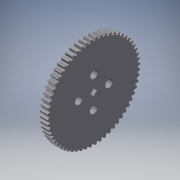
# Autodesk Inventor part: gear60
Saved by Autodesk Inventor 2019 (Build 230136000, 136)
## iProperties
Created: 2019-01-24
Part Number: gear60
Material: Generic
Document SubType Name: Modeling
Designer: Varga Daniel
Density: 1 g/cm^3
Appearance: Default
Author: Varga Daniel
Autodesk Inventor part; units mm, degrees
ref_plane "YZ Plane" through (0, 0, 0) normal (1, 0, 0) x (0, 1, 0)
ref_plane "XZ Plane" through (0, 0, 0) normal (0, 1, 0) x (-1, 0, 0)
ref_plane "XY Plane" through (0, 0, 0) normal (0, 0, 1) x (1, 0, 0)
sketch "Sketch1" plane through (0, 0, 0) normal (1, 0, 0) x (0, 1, 0)
  line L0 (1.5877, 28.5868) -> (1.4918, 28.6064)
  line L1 (1.4918, 28.6064) -> (1.2998, 28.6492)
  line L2 (1.2998, 28.6492) -> (0.9152, 28.7484)
  line L3 (0.9152, 28.7484) -> (0.53, 28.8645)
  line L4 (0.53, 28.8645) -> (0.1446, 28.9962)
  line L5 (0.1446, 28.9962) -> (0.0483, 29.0315)
  line L6 (0.0483, 29.0315) -> (0.0085, 30.0293)
  line L7 (0.0085, 30.0293) -> (0.1018, 30.0721)
  line L8 (0.1018, 30.0721) -> (0.4755, 30.234)
  line L9 (0.4755, 30.234) -> (0.8502, 30.3803)
  line L10 (0.8502, 30.3803) -> (1.2257, 30.5098)
  line L11 (1.2257, 30.5098) -> (1.4137, 30.5678)
  line L12 (1.4137, 30.5678) -> (1.5078, 30.5949)
  line L13 (1.5078, 30.5949) -> (1.521, 31.6473)
  line L14 (1.521, 31.6473) -> (1.4277, 31.6768)
  line L15 (1.4277, 31.6768) -> (1.2412, 31.7395)
  line L16 (1.2412, 31.7395) -> (0.869, 31.8784)
  line L17 (0.869, 31.8784) -> (0.4981, 32.034)
  line L18 (0.4981, 32.034) -> (0.1286, 32.2053)
  line L19 (0.1286, 32.2053) -> (0.0365, 32.2505)
  line L20 (0.0365, 32.2505) -> (0.1012, 33.247)
  line L21 (0.1012, 33.247) -> (0.1985, 33.2798)
  line L22 (0.1985, 33.2798) -> (0.587, 33.4018)
  line L23 (0.587, 33.4018) -> (0.975, 33.5081)
  line L24 (0.975, 33.5081) -> (1.362, 33.5977)
  line L25 (1.362, 33.5977) -> (1.555, 33.6356)
  line L26 (1.555, 33.6356) -> (1.6514, 33.6528)
  line L27 (1.6514, 33.6528) -> (1.7745, 34.6981)
  line L28 (1.7745, 34.6981) -> (1.6848, 34.7372)
  line L29 (1.6848, 34.7372) -> (1.5059, 34.819)
  line L30 (1.5059, 34.819) -> (1.1503, 34.996)
  line L31 (1.1503, 34.996) -> (0.7977, 35.1896)
  line L32 (0.7977, 35.1896) -> (0.4481, 35.3986)
  line L33 (0.4481, 35.3986) -> (0.3612, 35.4531)
  line L34 (0.3612, 35.4531) -> (0.5298, 36.4374)
  line L35 (0.5298, 36.4374) -> (0.6299, 36.4599)
  line L36 (0.6299, 36.4599) -> (1.0291, 36.5406)
  line L37 (1.0291, 36.5406) -> (1.4261, 36.6058)
  line L38 (1.4261, 36.6058) -> (1.8203, 36.6544)
  line L39 (1.8203, 36.6544) -> (2.0162, 36.672)
  line L40 (2.0162, 36.672) -> (2.1138, 36.679)
  line L41 (2.1138, 36.679) -> (2.3456, 37.7056)
  line L42 (2.3456, 37.7056) -> (2.2604, 37.7539)
  line L43 (2.2604, 37.7539) -> (2.0911, 37.8539)
  line L44 (2.0911, 37.8539) -> (1.7559, 38.0672)
  line L45 (1.7559, 38.0672) -> (1.4255, 38.2965)
  line L46 (1.4255, 38.2965) -> (1.0996, 38.5409)
  line L47 (1.0996, 38.5409) -> (1.0189, 38.6042)
  line L48 (1.0189, 38.6042) -> (1.2894, 39.5655)
  line L49 (1.2894, 39.5655) -> (1.3914, 39.5774)
  line L50 (1.3914, 39.5774) -> (1.7968, 39.6159)
  line L51 (1.7968, 39.6159) -> (2.1984, 39.6393)
  line L52 (2.1984, 39.6393) -> (2.5956, 39.6464)
  line L53 (2.5956, 39.6464) -> (2.7923, 39.6434)
  line L54 (2.7923, 39.6434) -> (2.8901, 39.6402)
  line L55 (2.8901, 39.6402) -> (3.2279, 40.637)
  line L56 (3.2279, 40.637) -> (3.1482, 40.6939)
  line L57 (3.1482, 40.6939) -> (2.9903, 40.8111)
  line L58 (2.9903, 40.8111) -> (2.6792, 41.0582)
  line L59 (2.6792, 41.0582) -> (2.3746, 41.3209)
  line L60 (2.3746, 41.3209) -> (2.0761, 41.5979)
  line L61 (2.0761, 41.5979) -> (2.0024, 41.6694)
  line L62 (2.0024, 41.6694) -> (2.372, 42.5971)
  line L63 (2.372, 42.5971) -> (2.4746, 42.5983)
  line L64 (2.4746, 42.5983) -> (2.8818, 42.5942)
  line L65 (2.8818, 42.5942) -> (3.2836, 42.5755)
  line L66 (3.2836, 42.5755) -> (3.6794, 42.541)
  line L67 (3.6794, 42.541) -> (3.8747, 42.5175)
  line L68 (3.8747, 42.5175) -> (3.9716, 42.5041)
  line L69 (3.9716, 42.5041) -> (4.4117, 43.4601)
  line L70 (4.4117, 43.4601) -> (4.3385, 43.525)
  line L71 (4.3385, 43.525) -> (4.1936, 43.6581)
  line L72 (4.1936, 43.6581) -> (3.9101, 43.9364)
  line L73 (3.9101, 43.9364) -> (3.6346, 44.2294)
  line L74 (3.6346, 44.2294) -> (3.3667, 44.5362)
  line L75 (3.3667, 44.5362) -> (3.3008, 44.6149)
  line L76 (3.3008, 44.6149) -> (3.7653, 45.4989)
  line L77 (3.7653, 45.4989) -> (3.8675, 45.4894)
  line L78 (3.8675, 45.4894) -> (4.2721, 45.4428)
  line L79 (4.2721, 45.4428) -> (4.6698, 45.3821)
  line L80 (4.6698, 45.3821) -> (5.0597, 45.3065)
  line L81 (5.0597, 45.3065) -> (5.2515, 45.2626)
  line L82 (5.2515, 45.2626) -> (5.3465, 45.2391)
  line L83 (5.3465, 45.2391) -> (5.8842, 46.1439)
  line L84 (5.8842, 46.1439) -> (5.8181, 46.2161)
  line L85 (5.8181, 46.2161) -> (5.688, 46.3637)
  line L86 (5.688, 46.3637) -> (5.4351, 46.67)
  line L87 (5.4351, 46.67) -> (5.1918, 46.9903)
  line L88 (5.1918, 46.9903) -> (4.9574, 47.3234)
  line L89 (4.9574, 47.3234) -> (4.9002, 47.4086)
  line L90 (4.9002, 47.4086) -> (5.4545, 48.2392)
  line L91 (5.4545, 48.2392) -> (5.5551, 48.219)
  line L92 (5.5551, 48.219) -> (5.9526, 48.1303)
  line L93 (5.9526, 48.1303) -> (6.3418, 48.0285)
  line L94 (6.3418, 48.0285) -> (6.7217, 47.9125)
  line L95 (6.7217, 47.9125) -> (6.9078, 47.8489)
  line L96 (6.9078, 47.8489) -> (6.9999, 47.8156)
  line L97 (6.9999, 47.8156) -> (7.6292, 48.6592)
  line L98 (7.6292, 48.6592) -> (7.571, 48.7379)
  line L99 (7.571, 48.7379) -> (7.457, 48.8982)
  line L100 (7.457, 48.8982) -> (7.2376, 49.2293)
  line L101 (7.2376, 49.2293) -> (7.029, 49.5733)
  line L102 (7.029, 49.5733) -> (6.8307, 49.9291)
  line L103 (6.8307, 49.9291) -> (6.7827, 50.0197)
  line L104 (6.7827, 50.0197) -> (7.4209, 50.7878)
  line L105 (7.4209, 50.7878) -> (7.5188, 50.7573)
  line L106 (7.5188, 50.7573) -> (7.9049, 50.6276)
  line L107 (7.9049, 50.6276) -> (8.2813, 50.4855)
  line L108 (8.2813, 50.4855) -> (8.647, 50.3305)
  line L109 (8.647, 50.3305) -> (8.8255, 50.2478)
  line L110 (8.8255, 50.2478) -> (8.9135, 50.2051)
  line L111 (8.9135, 50.2051) -> (9.6275, 50.9783)
  line L112 (9.6275, 50.9783) -> (9.5779, 51.0627)
  line L113 (9.5779, 51.0627) -> (9.4812, 51.2341)
  line L114 (9.4812, 51.2341) -> (9.2976, 51.5863)
  line L115 (9.2976, 51.5863) -> (9.1261, 51.9502)
  line L116 (9.1261, 51.9502) -> (8.9661, 52.3247)
  line L117 (8.9661, 52.3247) -> (8.9279, 52.4199)
  line L118 (8.9279, 52.4199) -> (9.6428, 53.1171)
  line L119 (9.6428, 53.1171) -> (9.7371, 53.0764)
  line L120 (9.7371, 53.0764) -> (10.1075, 52.9071)
  line L121 (10.1075, 52.9071) -> (10.4669, 52.7265)
  line L122 (10.4669, 52.7265) -> (10.8144, 52.5341)
  line L123 (10.8144, 52.5341) -> (10.9833, 52.4332)
  line L124 (10.9833, 52.4332) -> (11.0664, 52.3814)
  line L125 (11.0664, 52.3814) -> (11.8573, 53.0758)
  line L126 (11.8573, 53.0758) -> (11.8168, 53.1649)
  line L127 (11.8168, 53.1649) -> (11.7386, 53.3454)
  line L128 (11.7386, 53.3454) -> (11.5928, 53.7149)
  line L129 (11.5928, 53.7149) -> (11.4603, 54.0947)
  line L130 (11.4603, 54.0947) -> (11.3404, 54.484)
  line L131 (11.3404, 54.484) -> (11.3123, 54.5827)
  line L132 (11.3123, 54.5827) -> (12.0961, 55.2013)
  line L133 (12.0961, 55.2013) -> (12.1856, 55.151)
  line L134 (12.1856, 55.151) -> (12.5363, 54.9439)
  line L135 (12.5363, 54.9439) -> (12.8749, 54.7267)
  line L136 (12.8749, 54.7267) -> (13.2004, 54.4991)
  line L137 (13.2004, 54.4991) -> (13.3578, 54.381)
  line L138 (13.3578, 54.381) -> (13.435, 54.3209)
  line L139 (13.435, 54.3209) -> (14.2942, 54.9288)
  line L140 (14.2942, 54.9288) -> (14.2632, 55.0216)
  line L141 (14.2632, 55.0216) -> (14.2043, 55.2093)
  line L142 (14.2043, 55.2093) -> (14.0979, 55.592)
  line L143 (14.0979, 55.592) -> (14.0058, 55.9836)
  line L144 (14.0058, 55.9836) -> (13.9272, 56.3832)
  line L145 (13.9272, 56.3832) -> (13.9096, 56.4843)
  line L146 (13.9096, 56.4843) -> (14.7539, 57.0176)
  line L147 (14.7539, 57.0176) -> (14.8376, 56.9583)
  line L148 (14.8376, 56.9583) -> (15.1647, 56.7156)
  line L149 (15.1647, 56.7156) -> (15.4787, 56.4642)
  line L150 (15.4787, 56.4642) -> (15.7786, 56.2038)
  line L151 (15.7786, 56.2038) -> (15.9228, 56.07)
  line L152 (15.9228, 56.07) -> (15.9934, 56.0021)
  line L153 (15.9934, 56.0021) -> (16.9114, 56.5168)
  line L154 (16.9114, 56.5168) -> (16.8902, 56.6124)
  line L155 (16.8902, 56.6124) -> (16.8513, 56.8053)
  line L156 (16.8513, 56.8053) -> (16.7855, 57.197)
  line L157 (16.7855, 57.197) -> (16.7348, 57.596)
  line L158 (16.7348, 57.596) -> (16.6984, 58.0017)
  line L159 (16.6984, 58.0017) -> (16.6914, 58.1041)
  line L160 (16.6914, 58.1041) -> (17.5868, 58.5462)
  line L161 (17.5868, 58.5462) -> (17.6638, 58.4784)
  line L162 (17.6638, 58.4784) -> (17.9638, 58.2029)
  line L163 (17.9638, 58.2029) -> (18.2498, 57.9201)
  line L164 (18.2498, 57.9201) -> (18.5209, 57.6297)
  line L165 (18.5209, 57.6297) -> (18.6503, 57.4815)
  line L166 (18.6503, 57.4815) -> (18.7133, 57.4067)
  line L167 (18.7133, 57.4067) -> (19.6801, 57.8226)
  line L168 (19.6801, 57.8226) -> (19.6691, 57.9199)
  line L169 (19.6691, 57.9199) -> (19.6505, 58.1158)
  line L170 (19.6505, 58.1158) -> (19.626, 58.5122)
  line L171 (19.626, 58.5122) -> (19.6174, 58.9144)
  line L172 (19.6174, 58.9144) -> (19.6235, 59.3216)
  line L173 (19.6235, 59.3216) -> (19.6273, 59.4242)
  line L174 (19.6273, 59.4242) -> (20.564, 59.7703)
  line L175 (20.564, 59.7703) -> (20.6336, 59.6948)
  line L176 (20.6336, 59.6948) -> (20.9031, 59.3895)
  line L177 (20.9031, 59.3895) -> (21.158, 59.0783)
  line L178 (21.158, 59.0783) -> (21.3972, 58.7612)
  line L179 (21.3972, 58.7612) -> (21.5104, 58.6003)
  line L180 (21.5104, 58.6003) -> (21.5653, 58.5192)
  line L181 (21.5653, 58.5192) -> (22.5703, 58.8319)
  line L182 (22.5703, 58.8319) -> (22.5695, 58.9298)
  line L183 (22.5695, 58.9298) -> (22.5714, 59.1265)
  line L184 (22.5714, 59.1265) -> (22.5885, 59.5233)
  line L185 (22.5885, 59.5233) -> (22.622, 59.9242)
  line L186 (22.622, 59.9242) -> (22.6707, 60.3285)
  line L187 (22.6707, 60.3285) -> (22.6851, 60.4301)
  line L188 (22.6851, 60.4301) -> (23.6529, 60.6765)
  line L189 (23.6529, 60.6765) -> (23.7142, 60.5941)
  line L190 (23.7142, 60.5941) -> (23.9503, 60.2623)
  line L191 (23.9503, 60.2623) -> (24.1713, 59.9262)
  line L192 (24.1713, 59.9262) -> (24.376, 59.5858)
  line L193 (24.376, 59.5858) -> (24.4718, 59.4139)
  line L194 (24.4718, 59.4139) -> (24.5179, 59.3276)
  line L195 (24.5179, 59.3276) -> (25.55, 59.5335)
  line L196 (25.55, 59.5335) -> (25.5595, 59.6309)
  line L197 (25.5595, 59.6309) -> (25.582, 59.8263)
  line L198 (25.582, 59.8263) -> (25.6405, 60.2192)
  line L199 (25.6405, 60.2192) -> (25.7157, 60.6144)
  line L200 (25.7157, 60.6144) -> (25.8064, 61.0114)
  line L201 (25.8064, 61.0114) -> (25.8314, 61.111)
  line L202 (25.8314, 61.111) -> (26.8196, 61.2548)
  line L203 (26.8196, 61.2548) -> (26.8719, 61.1665)
  line L204 (26.8719, 61.1665) -> (27.072, 60.8118)
  line L205 (27.072, 60.8118) -> (27.2567, 60.4544)
  line L206 (27.2567, 60.4544) -> (27.4247, 60.0945)
  line L207 (27.4247, 60.0945) -> (27.502, 59.9136)
  line L208 (27.502, 59.9136) -> (27.5388, 59.8229)
  line L209 (27.5388, 59.8229) -> (28.5868, 59.9197)
  line L210 (28.5868, 59.9197) -> (28.6064, 60.0156)
  line L211 (28.6064, 60.0156) -> (28.6493, 60.2076)
  line L212 (28.6493, 60.2076) -> (28.7485, 60.5923)
  line L213 (28.7485, 60.5923) -> (28.8645, 60.9774)
  line L214 (28.8645, 60.9774) -> (28.9963, 61.3628)
  line L215 (28.9963, 61.3628) -> (29.0315, 61.4592)
  line L216 (29.0315, 61.4592) -> (30.0293, 61.4989)
  line L217 (30.0293, 61.4989) -> (30.0722, 61.4057)
  line L218 (30.0722, 61.4057) -> (30.2341, 61.0319)
  line L219 (30.2341, 61.0319) -> (30.3804, 60.6572)
  line L220 (30.3804, 60.6572) -> (30.5099, 60.2817)
  line L221 (30.5099, 60.2817) -> (30.5678, 60.0937)
  line L222 (30.5678, 60.0937) -> (30.595, 59.9997)
  line L223 (30.595, 59.9997) -> (31.6474, 59.9865)
  line L224 (31.6474, 59.9865) -> (31.6769, 60.0798)
  line L225 (31.6769, 60.0798) -> (31.7396, 60.2663)
  line L226 (31.7396, 60.2663) -> (31.8784, 60.6384)
  line L227 (31.8784, 60.6384) -> (32.0341, 61.0093)
  line L228 (32.0341, 61.0093) -> (32.2054, 61.3789)
  line L229 (32.2054, 61.3789) -> (32.2505, 61.471)
  line L230 (32.2505, 61.471) -> (33.247, 61.4062)
  line L231 (33.247, 61.4062) -> (33.2799, 61.309)
  line L232 (33.2799, 61.309) -> (33.4019, 60.9204)
  line L233 (33.4019, 60.9204) -> (33.5082, 60.5325)
  line L234 (33.5082, 60.5325) -> (33.5977, 60.1455)
  line L235 (33.5977, 60.1455) -> (33.6357, 59.9524)
  line L236 (33.6357, 59.9524) -> (33.6529, 59.8561)
  line L237 (33.6529, 59.8561) -> (34.6981, 59.7329)
  line L238 (34.6981, 59.7329) -> (34.7372, 59.8227)
  line L239 (34.7372, 59.8227) -> (34.8191, 60.0016)
  line L240 (34.8191, 60.0016) -> (34.9961, 60.3572)
  line L241 (34.9961, 60.3572) -> (35.1897, 60.7098)
  line L242 (35.1897, 60.7098) -> (35.3986, 61.0594)
  line L243 (35.3986, 61.0594) -> (35.4532, 61.1463)
  line L244 (35.4532, 61.1463) -> (36.4374, 60.9777)
  line L245 (36.4374, 60.9777) -> (36.4599, 60.8776)
  line L246 (36.4599, 60.8776) -> (36.5407, 60.4783)
  line L247 (36.5407, 60.4783) -> (36.6058, 60.0814)
  line L248 (36.6058, 60.0814) -> (36.6544, 59.6872)
  line L249 (36.6544, 59.6872) -> (36.672, 59.4912)
  line L250 (36.672, 59.4912) -> (36.679, 59.3936)
  line L251 (36.679, 59.3936) -> (37.7057, 59.1619)
  line L252 (37.7057, 59.1619) -> (37.754, 59.247)
  line L253 (37.754, 59.247) -> (37.854, 59.4164)
  line L254 (37.854, 59.4164) -> (38.0672, 59.7515)
  line L255 (38.0672, 59.7515) -> (38.2966, 60.082)
  line L256 (38.2966, 60.082) -> (38.541, 60.4078)
  line L257 (38.541, 60.4078) -> (38.6043, 60.4886)
  line L258 (38.6043, 60.4886) -> (39.5656, 60.218)
  line L259 (39.5656, 60.218) -> (39.5775, 60.1161)
  line L260 (39.5775, 60.1161) -> (39.616, 59.7106)
  line L261 (39.616, 59.7106) -> (39.6394, 59.309)
  line L262 (39.6394, 59.309) -> (39.6465, 58.9119)
  line L263 (39.6465, 58.9119) -> (39.6435, 58.7152)
  line L264 (39.6435, 58.7152) -> (39.6403, 58.6174)
  line L265 (39.6403, 58.6174) -> (40.6371, 58.2796)
  line L266 (40.6371, 58.2796) -> (40.694, 58.3592)
  line L267 (40.694, 58.3592) -> (40.8112, 58.5172)
  line L268 (40.8112, 58.5172) -> (41.0583, 58.8282)
  line L269 (41.0583, 58.8282) -> (41.3209, 59.1329)
  line L270 (41.3209, 59.1329) -> (41.598, 59.4314)
  line L271 (41.598, 59.4314) -> (41.6694, 59.5051)
  line L272 (41.6694, 59.5051) -> (42.5971, 59.1355)
  line L273 (42.5971, 59.1355) -> (42.5983, 59.0329)
  line L274 (42.5983, 59.0329) -> (42.5943, 58.6256)
  line L275 (42.5943, 58.6256) -> (42.5755, 58.2238)
  line L276 (42.5755, 58.2238) -> (42.5411, 57.8281)
  line L277 (42.5411, 57.8281) -> (42.5176, 57.6328)
  line L278 (42.5176, 57.6328) -> (42.5042, 57.5358)
  line L279 (42.5042, 57.5358) -> (43.4602, 57.0957)
  line L280 (43.4602, 57.0957) -> (43.5251, 57.169)
  line L281 (43.5251, 57.169) -> (43.6582, 57.3139)
  line L282 (43.6582, 57.3139) -> (43.9364, 57.5974)
  line L283 (43.9364, 57.5974) -> (44.2295, 57.8729)
  line L284 (44.2295, 57.8729) -> (44.5363, 58.1408)
  line L285 (44.5363, 58.1408) -> (44.615, 58.2066)
  line L286 (44.615, 58.2066) -> (45.499, 57.7421)
  line L287 (45.499, 57.7421) -> (45.4895, 57.64)
  line L288 (45.4895, 57.64) -> (45.4428, 57.2353)
  line L289 (45.4428, 57.2353) -> (45.3822, 56.8377)
  line L290 (45.3822, 56.8377) -> (45.3065, 56.4477)
  line L291 (45.3065, 56.4477) -> (45.2627, 56.2559)
  line L292 (45.2627, 56.2559) -> (45.2392, 56.1609)
  line L293 (45.2392, 56.1609) -> (46.144, 55.6233)
  line L294 (46.144, 55.6233) -> (46.2162, 55.6893)
  line L295 (46.2162, 55.6893) -> (46.3637, 55.8195)
  line L296 (46.3637, 55.8195) -> (46.6701, 56.0723)
  line L297 (46.6701, 56.0723) -> (46.9904, 56.3157)
  line L298 (46.9904, 56.3157) -> (47.3235, 56.5501)
  line L299 (47.3235, 56.5501) -> (47.4086, 56.6073)
  line L300 (47.4086, 56.6073) -> (48.2393, 56.053)
  line L301 (48.2393, 56.053) -> (48.2191, 55.9523)
  line L302 (48.2191, 55.9523) -> (48.1304, 55.5548)
  line L303 (48.1304, 55.5548) -> (48.0285, 55.1657)
  line L304 (48.0285, 55.1657) -> (47.9126, 54.7858)
  line L305 (47.9126, 54.7858) -> (47.849, 54.5996)
  line L306 (47.849, 54.5996) -> (47.8156, 54.5076)
  line L307 (47.8156, 54.5076) -> (48.6593, 53.8783)
  line L308 (48.6593, 53.8783) -> (48.738, 53.9364)
  line L309 (48.738, 53.9364) -> (48.8983, 54.0505)
  line L310 (48.8983, 54.0505) -> (49.2294, 54.2699)
  line L311 (49.2294, 54.2699) -> (49.5734, 54.4785)
  line L312 (49.5734, 54.4785) -> (49.9291, 54.6767)
  line L313 (49.9291, 54.6767) -> (50.0198, 54.7248)
  line L314 (50.0198, 54.7248) -> (50.7879, 54.0866)
  line L315 (50.7879, 54.0866) -> (50.7573, 53.9886)
  line L316 (50.7573, 53.9886) -> (50.6276, 53.6026)
  line L317 (50.6276, 53.6026) -> (50.4856, 53.2262)
  line L318 (50.4856, 53.2262) -> (50.3306, 52.8605)
  line L319 (50.3306, 52.8605) -> (50.2479, 52.682)
  line L320 (50.2479, 52.682) -> (50.2051, 52.5939)
  line L321 (50.2051, 52.5939) -> (50.9784, 51.88)
  line L322 (50.9784, 51.88) -> (51.0628, 51.9296)
  line L323 (51.0628, 51.9296) -> (51.2342, 52.0262)
  line L324 (51.2342, 52.0262) -> (51.5864, 52.2098)
  line L325 (51.5864, 52.2098) -> (51.9502, 52.3813)
  line L326 (51.9502, 52.3813) -> (52.3248, 52.5413)
  line L327 (52.3248, 52.5413) -> (52.42, 52.5796)
  line L328 (52.42, 52.5796) -> (53.1172, 51.8646)
  line L329 (53.1172, 51.8646) -> (53.0765, 51.7704)
  line L330 (53.0765, 51.7704) -> (52.9071, 51.4)
  line L331 (52.9071, 51.4) -> (52.7266, 51.0405)
  line L332 (52.7266, 51.0405) -> (52.5342, 50.693)
  line L333 (52.5342, 50.693) -> (52.4332, 50.5242)
  line L334 (52.4332, 50.5242) -> (52.3815, 50.4411)
  line L335 (52.3815, 50.4411) -> (53.0759, 49.6501)
  line L336 (53.0759, 49.6501) -> (53.165, 49.6907)
  line L337 (53.165, 49.6907) -> (53.3455, 49.7689)
  line L338 (53.3455, 49.7689) -> (53.715, 49.9147)
  line L339 (53.715, 49.9147) -> (54.0948, 50.0471)
  line L340 (54.0948, 50.0471) -> (54.484, 50.1671)
  line L341 (54.484, 50.1671) -> (54.5827, 50.1952)
  line L342 (54.5827, 50.1952) -> (55.2014, 49.4113)
  line L343 (55.2014, 49.4113) -> (55.1511, 49.3218)
  line L344 (55.1511, 49.3218) -> (54.944, 48.9712)
  line L345 (54.944, 48.9712) -> (54.7268, 48.6326)
  line L346 (54.7268, 48.6326) -> (54.4991, 48.3071)
  line L347 (54.4991, 48.3071) -> (54.3811, 48.1497)
  line L348 (54.3811, 48.1497) -> (54.321, 48.0725)
  line L349 (54.321, 48.0725) -> (54.9289, 47.2133)
  line L350 (54.9289, 47.2133) -> (55.0217, 47.2443)
  line L351 (55.0217, 47.2443) -> (55.2094, 47.3032)
  line L352 (55.2094, 47.3032) -> (55.5921, 47.4096)
  line L353 (55.5921, 47.4096) -> (55.9837, 47.5016)
  line L354 (55.9837, 47.5016) -> (56.3833, 47.5803)
  line L355 (56.3833, 47.5803) -> (56.4844, 47.5979)
  line L356 (56.4844, 47.5979) -> (57.0177, 46.7536)
  line L357 (57.0177, 46.7536) -> (56.9584, 46.6699)
  line L358 (56.9584, 46.6699) -> (56.7157, 46.3428)
  line L359 (56.7157, 46.3428) -> (56.4643, 46.0287)
  line L360 (56.4643, 46.0287) -> (56.2039, 45.7288)
  line L361 (56.2039, 45.7288) -> (56.07, 45.5847)
  line L362 (56.07, 45.5847) -> (56.0022, 45.5141)
  line L363 (56.0022, 45.5141) -> (56.5169, 44.5961)
  line L364 (56.5169, 44.5961) -> (56.6125, 44.6172)
  line L365 (56.6125, 44.6172) -> (56.8054, 44.6562)
  line L366 (56.8054, 44.6562) -> (57.1971, 44.722)
  line L367 (57.1971, 44.722) -> (57.5961, 44.7726)
  line L368 (57.5961, 44.7726) -> (58.0018, 44.8091)
  line L369 (58.0018, 44.8091) -> (58.1042, 44.8161)
  line L370 (58.1042, 44.8161) -> (58.5463, 43.9207)
  line L371 (58.5463, 43.9207) -> (58.4785, 43.8436)
  line L372 (58.4785, 43.8436) -> (58.203, 43.5437)
  line L373 (58.203, 43.5437) -> (57.9202, 43.2576)
  line L374 (57.9202, 43.2576) -> (57.6298, 42.9866)
  line L375 (57.6298, 42.9866) -> (57.4816, 42.8572)
  line L376 (57.4816, 42.8572) -> (57.4068, 42.7941)
  line L377 (57.4068, 42.7941) -> (57.8227, 41.8273)
  line L378 (57.8227, 41.8273) -> (57.92, 41.8383)
  line L379 (57.92, 41.8383) -> (58.1159, 41.8569)
  line L380 (58.1159, 41.8569) -> (58.5123, 41.8814)
  line L381 (58.5123, 41.8814) -> (58.9145, 41.8901)
  line L382 (58.9145, 41.8901) -> (59.3217, 41.8839)
  line L383 (59.3217, 41.8839) -> (59.4243, 41.8801)
  line L384 (59.4243, 41.8801) -> (59.7704, 40.9434)
  line L385 (59.7704, 40.9434) -> (59.6949, 40.8739)
  line L386 (59.6949, 40.8739) -> (59.3895, 40.6044)
  line L387 (59.3895, 40.6044) -> (59.0784, 40.3495)
  line L388 (59.0784, 40.3495) -> (58.7613, 40.1103)
  line L389 (58.7613, 40.1103) -> (58.6004, 39.997)
  line L390 (58.6004, 39.997) -> (58.5193, 39.9422)
  line L391 (58.5193, 39.9422) -> (58.832, 38.9372)
  line L392 (58.832, 38.9372) -> (58.9298, 38.938)
  line L393 (58.9298, 38.938) -> (59.1266, 38.936)
  line L394 (59.1266, 38.936) -> (59.5234, 38.9189)
  line L395 (59.5234, 38.9189) -> (59.9243, 38.8855)
  line L396 (59.9243, 38.8855) -> (60.3286, 38.8368)
  line L397 (60.3286, 38.8368) -> (60.4302, 38.8223)
  line L398 (60.4302, 38.8223) -> (60.6765, 37.8546)
  line L399 (60.6765, 37.8546) -> (60.5942, 37.7933)
  line L400 (60.5942, 37.7933) -> (60.2624, 37.5572)
  line L401 (60.2624, 37.5572) -> (59.9262, 37.3362)
  line L402 (59.9262, 37.3362) -> (59.5859, 37.1314)
  line L403 (59.5859, 37.1314) -> (59.414, 37.0357)
  line L404 (59.414, 37.0357) -> (59.3277, 36.9895)
  line L405 (59.3277, 36.9895) -> (59.5336, 35.9574)
  line L406 (59.5336, 35.9574) -> (59.631, 35.9479)
  line L407 (59.631, 35.9479) -> (59.8264, 35.9254)
  line L408 (59.8264, 35.9254) -> (60.2193, 35.8669)
  line L409 (60.2193, 35.8669) -> (60.6145, 35.7918)
  line L410 (60.6145, 35.7918) -> (61.0115, 35.7011)
  line L411 (61.0115, 35.7011) -> (61.1111, 35.6761)
  line L412 (61.1111, 35.6761) -> (61.2549, 34.6879)
  line L413 (61.2549, 34.6879) -> (61.166, 34.6351)
  line L414 (61.166, 34.6351) -> (60.8112, 34.435)
  line L415 (60.8112, 34.435) -> (60.4539, 34.2504)
  line L416 (60.4539, 34.2504) -> (60.0941, 34.0824)
  line L417 (60.0941, 34.0824) -> (59.9131, 34.0051)
  line L418 (59.9131, 34.0051) -> (59.8224, 33.9683)
  line L419 (59.8224, 33.9683) -> (59.9193, 32.9203)
  line L420 (59.9193, 32.9203) -> (60.016, 32.9005)
  line L421 (60.016, 32.9005) -> (60.208, 32.8577)
  line L422 (60.208, 32.8577) -> (60.5926, 32.7585)
  line L423 (60.5926, 32.7585) -> (60.9778, 32.6424)
  line L424 (60.9778, 32.6424) -> (61.3632, 32.5107)
  line L425 (61.3632, 32.5107) -> (61.4595, 32.4754)
  line L426 (61.4595, 32.4754) -> (61.4992, 31.4784)
  line L427 (61.4992, 31.4784) -> (61.4056, 31.4354)
  line L428 (61.4056, 31.4354) -> (61.0319, 31.2735)
  line L429 (61.0319, 31.2735) -> (60.6572, 31.1272)
  line L430 (60.6572, 31.1272) -> (60.2817, 30.9977)
  line L431 (60.2817, 30.9977) -> (60.0937, 30.9398)
  line L432 (60.0937, 30.9398) -> (59.9996, 30.9126)
  line L433 (59.9996, 30.9126) -> (59.9864, 29.8602)
  line L434 (59.9864, 29.8602) -> (60.0797, 29.8307)
  line L435 (60.0797, 29.8307) -> (60.2662, 29.768)
  line L436 (60.2662, 29.768) -> (60.6384, 29.6292)
  line L437 (60.6384, 29.6292) -> (61.0093, 29.4735)
  line L438 (61.0093, 29.4735) -> (61.3788, 29.3022)
  line L439 (61.3788, 29.3022) -> (61.4709, 29.2571)
  line L440 (61.4709, 29.2571) -> (61.4062, 28.2615)
  line L441 (61.4062, 28.2615) -> (61.3094, 28.2287)
  line L442 (61.3094, 28.2287) -> (60.9208, 28.1068)
  line L443 (60.9208, 28.1068) -> (60.5328, 28.0004)
  line L444 (60.5328, 28.0004) -> (60.1458, 27.9109)
  line L445 (60.1458, 27.9109) -> (59.9528, 27.8729)
  line L446 (59.9528, 27.8729) -> (59.8564, 27.8557)
  line L447 (59.8564, 27.8557) -> (59.7333, 26.8105)
  line L448 (59.7333, 26.8105) -> (59.823, 26.7714)
  line L449 (59.823, 26.7714) -> (60.0019, 26.6896)
  line L450 (60.0019, 26.6896) -> (60.3575, 26.5126)
  line L451 (60.3575, 26.5126) -> (60.7101, 26.319)
  line L452 (60.7101, 26.319) -> (61.0597, 26.11)
  line L453 (61.0597, 26.11) -> (61.1467, 26.0555)
  line L454 (61.1467, 26.0555) -> (60.9781, 25.0712)
  line L455 (60.9781, 25.0712) -> (60.8779, 25.0487)
  line L456 (60.8779, 25.0487) -> (60.4787, 24.968)
  line L457 (60.4787, 24.968) -> (60.0818, 24.9028)
  line L458 (60.0818, 24.9028) -> (59.6876, 24.8542)
  line L459 (59.6876, 24.8542) -> (59.4916, 24.8366)
  line L460 (59.4916, 24.8366) -> (59.394, 24.8296)
  line L461 (59.394, 24.8296) -> (59.1622, 23.8029)
  line L462 (59.1622, 23.8029) -> (59.2474, 23.7547)
  line L463 (59.2474, 23.7547) -> (59.4168, 23.6546)
  line L464 (59.4168, 23.6546) -> (59.7519, 23.4414)
  line L465 (59.7519, 23.4414) -> (60.0823, 23.212)
  line L466 (60.0823, 23.212) -> (60.4082, 22.9676)
  line L467 (60.4082, 22.9676) -> (60.4889, 22.9043)
  line L468 (60.4889, 22.9043) -> (60.2184, 21.9431)
  line L469 (60.2184, 21.9431) -> (60.1165, 21.9311)
  line L470 (60.1165, 21.9311) -> (59.711, 21.8926)
  line L471 (59.711, 21.8926) -> (59.3094, 21.8693)
  line L472 (59.3094, 21.8693) -> (58.9123, 21.8622)
  line L473 (58.9123, 21.8622) -> (58.7156, 21.8651)
  line L474 (58.7156, 21.8651) -> (58.6175, 21.8684)
  line L475 (58.6175, 21.8684) -> (58.2797, 20.8716)
  line L476 (58.2797, 20.8716) -> (58.3594, 20.8147)
  line L477 (58.3594, 20.8147) -> (58.5174, 20.6974)
  line L478 (58.5174, 20.6974) -> (58.8284, 20.4504)
  line L479 (58.8284, 20.4504) -> (59.133, 20.1877)
  line L480 (59.133, 20.1877) -> (59.4316, 19.9106)
  line L481 (59.4316, 19.9106) -> (59.5052, 19.8392)
  line L482 (59.5052, 19.8392) -> (59.1357, 18.9115)
  line L483 (59.1357, 18.9115) -> (59.0331, 18.9103)
  line L484 (59.0331, 18.9103) -> (58.6258, 18.9143)
  line L485 (58.6258, 18.9143) -> (58.224, 18.9331)
  line L486 (58.224, 18.9331) -> (57.8283, 18.9675)
  line L487 (57.8283, 18.9675) -> (57.6329, 18.991)
  line L488 (57.6329, 18.991) -> (57.536, 19.0045)
  line L489 (57.536, 19.0045) -> (57.0955, 18.0476)
  line L490 (57.0955, 18.0476) -> (57.1691, 17.9823)
  line L491 (57.1691, 17.9823) -> (57.314, 17.8493)
  line L492 (57.314, 17.8493) -> (57.5975, 17.571)
  line L493 (57.5975, 17.571) -> (57.873, 17.278)
  line L494 (57.873, 17.278) -> (58.1409, 16.9712)
  line L495 (58.1409, 16.9712) -> (58.2067, 16.8925)
  line L496 (58.2067, 16.8925) -> (57.7422, 16.0085)
  line L497 (57.7422, 16.0085) -> (57.6401, 16.018)
  line L498 (57.6401, 16.018) -> (57.2355, 16.0646)
  line L499 (57.2355, 16.0646) -> (56.8378, 16.1253)
  line L500 (56.8378, 16.1253) -> (56.4479, 16.2009)
  line L501 (56.4479, 16.2009) -> (56.2561, 16.2447)
  line L502 (56.2561, 16.2447) -> (56.161, 16.2682)
  line L503 (56.161, 16.2682) -> (55.6234, 15.3635)
  line L504 (55.6234, 15.3635) -> (55.6895, 15.2912)
  line L505 (55.6895, 15.2912) -> (55.8196, 15.1437)
  line L506 (55.8196, 15.1437) -> (56.0724, 14.8374)
  line L507 (56.0724, 14.8374) -> (56.3158, 14.5171)
  line L508 (56.3158, 14.5171) -> (56.5502, 14.184)
  line L509 (56.5502, 14.184) -> (56.6074, 14.0988)
  line L510 (56.6074, 14.0988) -> (56.0531, 13.2682)
  line L511 (56.0531, 13.2682) -> (55.9525, 13.2884)
  line L512 (55.9525, 13.2884) -> (55.5549, 13.377)
  line L513 (55.5549, 13.377) -> (55.1658, 13.4789)
  line L514 (55.1658, 13.4789) -> (54.7859, 13.5949)
  line L515 (54.7859, 13.5949) -> (54.5997, 13.6585)
  line L516 (54.5997, 13.6585) -> (54.5077, 13.6918)
  line L517 (54.5077, 13.6918) -> (53.8784, 12.8482)
  line L518 (53.8784, 12.8482) -> (53.9366, 12.7695)
  line L519 (53.9366, 12.7695) -> (54.0506, 12.6092)
  line L520 (54.0506, 12.6092) -> (54.27, 12.2781)
  line L521 (54.27, 12.2781) -> (54.4786, 11.9341)
  line L522 (54.4786, 11.9341) -> (54.6769, 11.5783)
  line L523 (54.6769, 11.5783) -> (54.7249, 11.4876)
  line L524 (54.7249, 11.4876) -> (54.0867, 10.7196)
  line L525 (54.0867, 10.7196) -> (53.9888, 10.7501)
  line L526 (53.9888, 10.7501) -> (53.6027, 10.8798)
  line L527 (53.6027, 10.8798) -> (53.2263, 11.0218)
  line L528 (53.2263, 11.0218) -> (52.8606, 11.1769)
  line L529 (52.8606, 11.1769) -> (52.6821, 11.2596)
  line L530 (52.6821, 11.2596) -> (52.5941, 11.3023)
  line L531 (52.5941, 11.3023) -> (51.8801, 10.529)
  line L532 (51.8801, 10.529) -> (51.9297, 10.4447)
  line L533 (51.9297, 10.4447) -> (52.0264, 10.2733)
  line L534 (52.0264, 10.2733) -> (52.21, 9.9211)
  line L535 (52.21, 9.9211) -> (52.3815, 9.5572)
  line L536 (52.3815, 9.5572) -> (52.5414, 9.1827)
  line L537 (52.5414, 9.1827) -> (52.5797, 9.0874)
  line L538 (52.5797, 9.0874) -> (51.8648, 8.3903)
  line L539 (51.8648, 8.3903) -> (51.7705, 8.4309)
  line L540 (51.7705, 8.4309) -> (51.4001, 8.6003)
  line L541 (51.4001, 8.6003) -> (51.0407, 8.7809)
  line L542 (51.0407, 8.7809) -> (50.6932, 8.9733)
  line L543 (50.6932, 8.9733) -> (50.5243, 9.0742)
  line L544 (50.5243, 9.0742) -> (50.4412, 9.1259)
  line L545 (50.4412, 9.1259) -> (49.6503, 8.4316)
  line L546 (49.6503, 8.4316) -> (49.6908, 8.3425)
  line L547 (49.6908, 8.3425) -> (49.769, 8.162)
  line L548 (49.769, 8.162) -> (49.9148, 7.7925)
  line L549 (49.9148, 7.7925) -> (50.0473, 7.4126)
  line L550 (50.0473, 7.4126) -> (50.1672, 7.0234)
  line L551 (50.1672, 7.0234) -> (50.1953, 6.9247)
  line L552 (50.1953, 6.9247) -> (49.4114, 6.3061)
  line L553 (49.4114, 6.3061) -> (49.322, 6.3563)
  line L554 (49.322, 6.3563) -> (48.9713, 6.5635)
  line L555 (48.9713, 6.5635) -> (48.6327, 6.7806)
  line L556 (48.6327, 6.7806) -> (48.3072, 7.0083)
  line L557 (48.3072, 7.0083) -> (48.1498, 7.1264)
  line L558 (48.1498, 7.1264) -> (48.0726, 7.1865)
  line L559 (48.0726, 7.1865) -> (47.2134, 6.5786)
  line L560 (47.2134, 6.5786) -> (47.2444, 6.4857)
  line L561 (47.2444, 6.4857) -> (47.3033, 6.298)
  line L562 (47.3033, 6.298) -> (47.4097, 5.9153)
  line L563 (47.4097, 5.9153) -> (47.5018, 5.5238)
  line L564 (47.5018, 5.5238) -> (47.5804, 5.1241)
  line L565 (47.5804, 5.1241) -> (47.598, 5.023)
  line L566 (47.598, 5.023) -> (46.7537, 4.4897)
  line L567 (46.7537, 4.4897) -> (46.67, 4.5491)
  line L568 (46.67, 4.5491) -> (46.3429, 4.7918)
  line L569 (46.3429, 4.7918) -> (46.0289, 5.0431)
  line L570 (46.0289, 5.0431) -> (45.729, 5.3036)
  line L571 (45.729, 5.3036) -> (45.5848, 5.4374)
  line L572 (45.5848, 5.4374) -> (45.5142, 5.5053)
  line L573 (45.5142, 5.5053) -> (44.5962, 4.9905)
  line L574 (44.5962, 4.9905) -> (44.6173, 4.8949)
  line L575 (44.6173, 4.8949) -> (44.6563, 4.7021)
  line L576 (44.6563, 4.7021) -> (44.7221, 4.3104)
  line L577 (44.7221, 4.3104) -> (44.7728, 3.9113)
  line L578 (44.7728, 3.9113) -> (44.8092, 3.5057)
  line L579 (44.8092, 3.5057) -> (44.8162, 3.4033)
  line L580 (44.8162, 3.4033) -> (43.9208, 2.9611)
  line L581 (43.9208, 2.9611) -> (43.8437, 3.0289)
  line L582 (43.8437, 3.0289) -> (43.5438, 3.3045)
  line L583 (43.5438, 3.3045) -> (43.2577, 3.5873)
  line L584 (43.2577, 3.5873) -> (42.9867, 3.8776)
  line L585 (42.9867, 3.8776) -> (42.8573, 4.0258)
  line L586 (42.8573, 4.0258) -> (42.7942, 4.1007)
  line L587 (42.7942, 4.1007) -> (41.8274, 3.6847)
  line L588 (41.8274, 3.6847) -> (41.8384, 3.5875)
  line L589 (41.8384, 3.5875) -> (41.857, 3.3916)
  line L590 (41.857, 3.3916) -> (41.8815, 2.9952)
  line L591 (41.8815, 2.9952) -> (41.8902, 2.593)
  line L592 (41.8902, 2.593) -> (41.884, 2.1857)
  line L593 (41.884, 2.1857) -> (41.8802, 2.0832)
  line L594 (41.8802, 2.0832) -> (40.9435, 1.7371)
  line L595 (40.9435, 1.7371) -> (40.874, 1.8125)
  line L596 (40.874, 1.8125) -> (40.6045, 2.1179)
  line L597 (40.6045, 2.1179) -> (40.3496, 2.4291)
  line L598 (40.3496, 2.4291) -> (40.1104, 2.7462)
  line L599 (40.1104, 2.7462) -> (39.9972, 2.9071)
  line L600 (39.9972, 2.9071) -> (39.9423, 2.9881)
  line L601 (39.9423, 2.9881) -> (38.9373, 2.6755)
  line L602 (38.9373, 2.6755) -> (38.9381, 2.5776)
  line L603 (38.9381, 2.5776) -> (38.9361, 2.3809)
  line L604 (38.9361, 2.3809) -> (38.919, 1.984)
  line L605 (38.919, 1.984) -> (38.8856, 1.5832)
  line L606 (38.8856, 1.5832) -> (38.8369, 1.1788)
  line L607 (38.8369, 1.1788) -> (38.8224, 1.0772)
  line L608 (38.8224, 1.0772) -> (37.8547, 0.8309)
  line L609 (37.8547, 0.8309) -> (37.7934, 0.9132)
  line L610 (37.7934, 0.9132) -> (37.5573, 1.2451)
  line L611 (37.5573, 1.2451) -> (37.3363, 1.5812)
  line L612 (37.3363, 1.5812) -> (37.1316, 1.9216)
  line L613 (37.1316, 1.9216) -> (37.0358, 2.0934)
  line L614 (37.0358, 2.0934) -> (36.9897, 2.1798)
  line L615 (36.9897, 2.1798) -> (35.9575, 1.9739)
  line L616 (35.9575, 1.9739) -> (35.9481, 1.8765)
  line L617 (35.9481, 1.8765) -> (35.9255, 1.681)
  line L618 (35.9255, 1.681) -> (35.8671, 1.2882)
  line L619 (35.8671, 1.2882) -> (35.7919, 0.893)
  line L620 (35.7919, 0.893) -> (35.7012, 0.4959)
  line L621 (35.7012, 0.4959) -> (35.6762, 0.3964)
  line L622 (35.6762, 0.3964) -> (34.688, 0.2526)
  line L623 (34.688, 0.2526) -> (34.6357, 0.3408)
  line L624 (34.6357, 0.3408) -> (34.4355, 0.6956)
  line L625 (34.4355, 0.6956) -> (34.2509, 1.053)
  line L626 (34.2509, 1.053) -> (34.0828, 1.4129)
  line L627 (34.0828, 1.4129) -> (34.0056, 1.5938)
  line L628 (34.0056, 1.5938) -> (33.9687, 1.6845)
  line L629 (33.9687, 1.6845) -> (32.9207, 1.5876)
  line L630 (32.9207, 1.5876) -> (32.9011, 1.4917)
  line L631 (32.9011, 1.4917) -> (32.8583, 1.2997)
  line L632 (32.8583, 1.2997) -> (32.7591, 0.9151)
  line L633 (32.7591, 0.9151) -> (32.643, 0.5299)
  line L634 (32.643, 0.5299) -> (32.5113, 0.1445)
  line L635 (32.5113, 0.1445) -> (32.476, 0.0482)
  line L636 (32.476, 0.0482) -> (31.4782, 0.0084)
  line L637 (31.4782, 0.0084) -> (31.4354, 0.1017)
  line L638 (31.4354, 0.1017) -> (31.2735, 0.4754)
  line L639 (31.2735, 0.4754) -> (31.1272, 0.8501)
  line L640 (31.1272, 0.8501) -> (30.9977, 1.2256)
  line L641 (30.9977, 1.2256) -> (30.9397, 1.4136)
  line L642 (30.9397, 1.4136) -> (30.9126, 1.5077)
  line L643 (30.9126, 1.5077) -> (29.8602, 1.5209)
  line L644 (29.8602, 1.5209) -> (29.8307, 1.4276)
  line L645 (29.8307, 1.4276) -> (29.768, 1.2411)
  line L646 (29.768, 1.2411) -> (29.6291, 0.8689)
  line L647 (29.6291, 0.8689) -> (29.4735, 0.498)
  line L648 (29.4735, 0.498) -> (29.3022, 0.1285)
  line L649 (29.3022, 0.1285) -> (29.257, 0.0364)
  line L650 (29.257, 0.0364) -> (28.2605, 0.1011)
  line L651 (28.2605, 0.1011) -> (28.2277, 0.1984)
  line L652 (28.2277, 0.1984) -> (28.1057, 0.587)
  line L653 (28.1057, 0.587) -> (27.9994, 0.9749)
  line L654 (27.9994, 0.9749) -> (27.9098, 1.3619)
  line L655 (27.9098, 1.3619) -> (27.8718, 1.5549)
  line L656 (27.8718, 1.5549) -> (27.8547, 1.6513)
  line L657 (27.8547, 1.6513) -> (26.8094, 1.7744)
  line L658 (26.8094, 1.7744) -> (26.7703, 1.6847)
  line L659 (26.7703, 1.6847) -> (26.6885, 1.5058)
  line L660 (26.6885, 1.5058) -> (26.5115, 1.1502)
  line L661 (26.5115, 1.1502) -> (26.3179, 0.7976)
  line L662 (26.3179, 0.7976) -> (26.1089, 0.448)
  line L663 (26.1089, 0.448) -> (26.0544, 0.3611)
  line L664 (26.0544, 0.3611) -> (25.0701, 0.5297)
  line L665 (25.0701, 0.5297) -> (25.0476, 0.6298)
  line L666 (25.0476, 0.6298) -> (24.9669, 1.029)
  line L667 (24.9669, 1.029) -> (24.9017, 1.426)
  line L668 (24.9017, 1.426) -> (24.8531, 1.8202)
  line L669 (24.8531, 1.8202) -> (24.8355, 2.0161)
  line L670 (24.8355, 2.0161) -> (24.8285, 2.1138)
  line L671 (24.8285, 2.1138) -> (23.8019, 2.3455)
  line L672 (23.8019, 2.3455) -> (23.7536, 2.2603)
  line L673 (23.7536, 2.2603) -> (23.6535, 2.091)
  line L674 (23.6535, 2.091) -> (23.4403, 1.7558)
  line L675 (23.4403, 1.7558) -> (23.2109, 1.4254)
  line L676 (23.2109, 1.4254) -> (22.9666, 1.0996)
  line L677 (22.9666, 1.0996) -> (22.9032, 1.0188)
  line L678 (22.9032, 1.0188) -> (21.942, 1.2894)
  line L679 (21.942, 1.2894) -> (21.9301, 1.3913)
  line L680 (21.9301, 1.3913) -> (21.8915, 1.7967)
  line L681 (21.8915, 1.7967) -> (21.8682, 2.1983)
  line L682 (21.8682, 2.1983) -> (21.8611, 2.5955)
  line L683 (21.8611, 2.5955) -> (21.8641, 2.7922)
  line L684 (21.8641, 2.7922) -> (21.8673, 2.89)
  line L685 (21.8673, 2.89) -> (20.8705, 3.2278)
  line L686 (20.8705, 3.2278) -> (20.8136, 3.1481)
  line L687 (20.8136, 3.1481) -> (20.6964, 2.9902)
  line L688 (20.6964, 2.9902) -> (20.4493, 2.6791)
  line L689 (20.4493, 2.6791) -> (20.1866, 2.3745)
  line L690 (20.1866, 2.3745) -> (19.9095, 2.076)
  line L691 (19.9095, 2.076) -> (19.8381, 2.0023)
  line L692 (19.8381, 2.0023) -> (18.9104, 2.3719)
  line L693 (18.9104, 2.3719) -> (18.9092, 2.4745)
  line L694 (18.9092, 2.4745) -> (18.9133, 2.8817)
  line L695 (18.9133, 2.8817) -> (18.932, 3.2836)
  line L696 (18.932, 3.2836) -> (18.9664, 3.6793)
  line L697 (18.9664, 3.6793) -> (18.99, 3.8746)
  line L698 (18.99, 3.8746) -> (19.0034, 3.9716)
  line L699 (19.0034, 3.9716) -> (18.0473, 4.4116)
  line L700 (18.0473, 4.4116) -> (17.9824, 4.3384)
  line L701 (17.9824, 4.3384) -> (17.8493, 4.1935)
  line L702 (17.8493, 4.1935) -> (17.5711, 3.91)
  line L703 (17.5711, 3.91) -> (17.278, 3.6345)
  line L704 (17.278, 3.6345) -> (16.9713, 3.3666)
  line L705 (16.9713, 3.3666) -> (16.8925, 3.3008)
  line L706 (16.8925, 3.3008) -> (16.0085, 3.7653)
  line L707 (16.0085, 3.7653) -> (16.0181, 3.8674)
  line L708 (16.0181, 3.8674) -> (16.0647, 4.2721)
  line L709 (16.0647, 4.2721) -> (16.1254, 4.6697)
  line L710 (16.1254, 4.6697) -> (16.201, 5.0596)
  line L711 (16.201, 5.0596) -> (16.2448, 5.2514)
  line L712 (16.2448, 5.2514) -> (16.2683, 5.3465)
  line L713 (16.2683, 5.3465) -> (15.3635, 5.8841)
  line L714 (15.3635, 5.8841) -> (15.2913, 5.8181)
  line L715 (15.2913, 5.8181) -> (15.1438, 5.6879)
  line L716 (15.1438, 5.6879) -> (14.8374, 5.4351)
  line L717 (14.8374, 5.4351) -> (14.5172, 5.1917)
  line L718 (14.5172, 5.1917) -> (14.1841, 4.9573)
  line L719 (14.1841, 4.9573) -> (14.0989, 4.9001)
  line L720 (14.0989, 4.9001) -> (13.2683, 5.4544)
  line L721 (13.2683, 5.4544) -> (13.2885, 5.555)
  line L722 (13.2885, 5.555) -> (13.3771, 5.9526)
  line L723 (13.3771, 5.9526) -> (13.479, 6.3417)
  line L724 (13.479, 6.3417) -> (13.595, 6.7216)
  line L725 (13.595, 6.7216) -> (13.6586, 6.9078)
  line L726 (13.6586, 6.9078) -> (13.6919, 6.9998)
  line L727 (13.6919, 6.9998) -> (12.8483, 7.6291)
  line L728 (12.8483, 7.6291) -> (12.7695, 7.5709)
  line L729 (12.7695, 7.5709) -> (12.6092, 7.4569)
  line L730 (12.6092, 7.4569) -> (12.2781, 7.2375)
  line L731 (12.2781, 7.2375) -> (11.9342, 7.0289)
  line L732 (11.9342, 7.0289) -> (11.5784, 6.8306)
  line L733 (11.5784, 6.8306) -> (11.4877, 6.7826)
  line L734 (11.4877, 6.7826) -> (10.7196, 7.4208)
  line L735 (10.7196, 7.4208) -> (10.7502, 7.5187)
  line L736 (10.7502, 7.5187) -> (10.8799, 7.9048)
  line L737 (10.8799, 7.9048) -> (11.0219, 8.2812)
  line L738 (11.0219, 8.2812) -> (11.1769, 8.6469)
  line L739 (11.1769, 8.6469) -> (11.2597, 8.8254)
  line L740 (11.2597, 8.8254) -> (11.3024, 8.9135)
  line L741 (11.3024, 8.9135) -> (10.5291, 9.6274)
  line L742 (10.5291, 9.6274) -> (10.4447, 9.5778)
  line L743 (10.4447, 9.5778) -> (10.2734, 9.4811)
  line L744 (10.2734, 9.4811) -> (9.9212, 9.2975)
  line L745 (9.9212, 9.2975) -> (9.5573, 9.126)
  line L746 (9.5573, 9.126) -> (9.1827, 8.9661)
  line L747 (9.1827, 8.9661) -> (9.0875, 8.9278)
  line L748 (9.0875, 8.9278) -> (8.3904, 9.6428)
  line L749 (8.3904, 9.6428) -> (8.431, 9.737)
  line L750 (8.431, 9.737) -> (8.6004, 10.1074)
  line L751 (8.6004, 10.1074) -> (8.781, 10.4668)
  line L752 (8.781, 10.4668) -> (8.9734, 10.8143)
  line L753 (8.9734, 10.8143) -> (9.0743, 10.9832)
  line L754 (9.0743, 10.9832) -> (9.126, 11.0663)
  line L755 (9.126, 11.0663) -> (8.4316, 11.8572)
  line L756 (8.4316, 11.8572) -> (8.3425, 11.8167)
  line L757 (8.3425, 11.8167) -> (8.162, 11.7385)
  line L758 (8.162, 11.7385) -> (7.7925, 11.5927)
  line L759 (7.7925, 11.5927) -> (7.4127, 11.4602)
  line L760 (7.4127, 11.4602) -> (7.0235, 11.3403)
  line L761 (7.0235, 11.3403) -> (6.9248, 11.3122)
  line L762 (6.9248, 11.3122) -> (6.3062, 12.0961)
  line L763 (6.3062, 12.0961) -> (6.3564, 12.1855)
  line L764 (6.3564, 12.1855) -> (6.5636, 12.5362)
  line L765 (6.5636, 12.5362) -> (6.7807, 12.8748)
  line L766 (6.7807, 12.8748) -> (7.0084, 13.2003)
  line L767 (7.0084, 13.2003) -> (7.1264, 13.3577)
  line L768 (7.1264, 13.3577) -> (7.1866, 13.4349)
  line L769 (7.1866, 13.4349) -> (6.5787, 14.2941)
  line L770 (6.5787, 14.2941) -> (6.4858, 14.2631)
  line L771 (6.4858, 14.2631) -> (6.2981, 14.2042)
  line L772 (6.2981, 14.2042) -> (5.9154, 14.0978)
  line L773 (5.9154, 14.0978) -> (5.5238, 14.0058)
  line L774 (5.5238, 14.0058) -> (5.1242, 13.9271)
  line L775 (5.1242, 13.9271) -> (5.0231, 13.9095)
  line L776 (5.0231, 13.9095) -> (4.4898, 14.7538)
  line L777 (4.4898, 14.7538) -> (4.5492, 14.8375)
  line L778 (4.5492, 14.8375) -> (4.7919, 15.1646)
  line L779 (4.7919, 15.1646) -> (5.0432, 15.4786)
  line L780 (5.0432, 15.4786) -> (5.3037, 15.7785)
  line L781 (5.3037, 15.7785) -> (5.4375, 15.9227)
  line L782 (5.4375, 15.9227) -> (5.5054, 15.9933)
  line L783 (5.5054, 15.9933) -> (4.9906, 16.9113)
  line L784 (4.9906, 16.9113) -> (4.895, 16.8902)
  line L785 (4.895, 16.8902) -> (4.7022, 16.8512)
  line L786 (4.7022, 16.8512) -> (4.3105, 16.7854)
  line L787 (4.3105, 16.7854) -> (3.9114, 16.7347)
  line L788 (3.9114, 16.7347) -> (3.5058, 16.6983)
  line L789 (3.5058, 16.6983) -> (3.4034, 16.6913)
  line L790 (3.4034, 16.6913) -> (2.9612, 17.5867)
  line L791 (2.9612, 17.5867) -> (3.029, 17.6638)
  line L792 (3.029, 17.6638) -> (3.3045, 17.9637)
  line L793 (3.3045, 17.9637) -> (3.5874, 18.2498)
  line L794 (3.5874, 18.2498) -> (3.8777, 18.5208)
  line L795 (3.8777, 18.5208) -> (4.0259, 18.6502)
  line L796 (4.0259, 18.6502) -> (4.1008, 18.7133)
  line L797 (4.1008, 18.7133) -> (3.6848, 19.6801)
  line L798 (3.6848, 19.6801) -> (3.5875, 19.6691)
  line L799 (3.5875, 19.6691) -> (3.3917, 19.6504)
  line L800 (3.3917, 19.6504) -> (2.9952, 19.626)
  line L801 (2.9952, 19.626) -> (2.5931, 19.6173)
  line L802 (2.5931, 19.6173) -> (2.1858, 19.6235)
  line L803 (2.1858, 19.6235) -> (2.0833, 19.6273)
  line L804 (2.0833, 19.6273) -> (1.7372, 20.5639)
  line L805 (1.7372, 20.5639) -> (1.8126, 20.6335)
  line L806 (1.8126, 20.6335) -> (2.118, 20.903)
  line L807 (2.118, 20.903) -> (2.4292, 21.1579)
  line L808 (2.4292, 21.1579) -> (2.7463, 21.3971)
  line L809 (2.7463, 21.3971) -> (2.9072, 21.5103)
  line L810 (2.9072, 21.5103) -> (2.9882, 21.5652)
  line L811 (2.9882, 21.5652) -> (2.6756, 22.5702)
  line L812 (2.6756, 22.5702) -> (2.5777, 22.5694)
  line L813 (2.5777, 22.5694) -> (2.381, 22.5714)
  line L814 (2.381, 22.5714) -> (1.9841, 22.5885)
  line L815 (1.9841, 22.5885) -> (1.5833, 22.6219)
  line L816 (1.5833, 22.6219) -> (1.1789, 22.6706)
  line L817 (1.1789, 22.6706) -> (1.0773, 22.6851)
  line L818 (1.0773, 22.6851) -> (0.831, 23.6528)
  line L819 (0.831, 23.6528) -> (0.9133, 23.7141)
  line L820 (0.9133, 23.7141) -> (1.2452, 23.9502)
  line L821 (1.2452, 23.9502) -> (1.5813, 24.1712)
  line L822 (1.5813, 24.1712) -> (1.9217, 24.3759)
  line L823 (1.9217, 24.3759) -> (2.0935, 24.4717)
  line L824 (2.0935, 24.4717) -> (2.1799, 24.5178)
  line L825 (2.1799, 24.5178) -> (1.974, 25.55)
  line L826 (1.974, 25.55) -> (1.8766, 25.5594)
  line L827 (1.8766, 25.5594) -> (1.6811, 25.5819)
  line L828 (1.6811, 25.5819) -> (1.2882, 25.6404)
  line L829 (1.2882, 25.6404) -> (0.8931, 25.7156)
  line L830 (0.8931, 25.7156) -> (0.496, 25.8063)
  line L831 (0.496, 25.8063) -> (0.3965, 25.8313)
  line L832 (0.3965, 25.8313) -> (0.2527, 26.8195)
  line L833 (0.2527, 26.8195) -> (0.3409, 26.8718)
  line L834 (0.3409, 26.8718) -> (0.6957, 27.0719)
  line L835 (0.6957, 27.0719) -> (1.0531, 27.2566)
  line L836 (1.0531, 27.2566) -> (1.413, 27.4246)
  line L837 (1.413, 27.4246) -> (1.5939, 27.5019)
  line L838 (1.5939, 27.5019) -> (1.6846, 27.5388)
  line L839 (1.6846, 27.5388) -> (1.5877, 28.5868)
  circle A0 centre (30.7537, 30.7537) radius 0.5
  line L840 (20.5024, 30.7537) -> (41.0049, 30.7537)
  line L841 (30.7537, 20.5024) -> (30.7537, 41.0049)
  point P0 (0, 0)
  constraints: 1684 end point, 425 perpendicular, 232 parallel, 1 centre point
extrude "Extrusion1" add sketch "Sketch1" along normal blind 5
sketch "Sketch6" plane through (5, 0, 0) normal (1, 0, 0) x (0, 0, -1)
  circle A0 centre (-40.7529, 30.8797) radius 2.45 projected
  circle A1 centre (-20.7545, 30.6276) radius 2.45 projected
  arc A2 (-30.9218, 28.6343) -> (-30.639, 28.6307) centre (-30.7786, 28.7739) ccw projected
  line L0 (-30.9218, 28.6343) -> (-32.8766, 30.639) projected
  arc A3 (-32.873, 30.9218) -> (-32.8766, 30.639) centre (-32.7334, 30.7786) ccw projected
  line L1 (-32.873, 30.9218) -> (-30.8683, 32.8766) projected
  arc A4 (-30.5855, 32.873) -> (-30.8683, 32.8766) centre (-30.7287, 32.7334) ccw projected
  line L2 (-30.5855, 32.873) -> (-28.6307, 30.8683) projected
  arc A5 (-28.6343, 30.5855) -> (-28.6307, 30.8683) centre (-28.7739, 30.7287) ccw projected
  line L3 (-28.6343, 30.5855) -> (-30.639, 28.6307) projected
  circle A6 centre (-30.6276, 40.7529) radius 2.45 projected
  circle A7 centre (-30.8797, 20.7545) radius 2.45 projected
  circle A8 centre (-30.7537, 30.7537) radius 15 projected
  point P0 (0, 0)
extrude "Extrusion6" cut sketch "Sketch6" against normal up to next contours A0 | A1 | L0 A3 L1 A4 L2 A5 L3 A2 | A6 | A7
body "Solid1"
